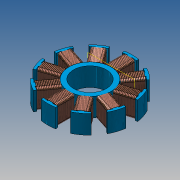
# Autodesk Inventor part: Coil
Saved by Autodesk Inventor 2015 (Build 190159000, 159)
## iProperties
Created: 2016-12-08
Part Number: Coil
Material: Allgemein
Document SubType Name: Modeling
Designer: NS
Density: 1 g/cm^3
Appearance: Default
RuleStatus: InUse
BeforeDocSave0: file://C:\_Vault_ausgecheckt\ilogic\ipt
Author: NS
Autodesk Inventor part; units mm, degrees
ref_plane "YZ Plane" through (0, 0, 0) normal (1, 0, 0) x (0, 1, 0)
ref_plane "XY Plane" through (0, 0, 0) normal (0, 0, 1) x (1, 0, 0)
sketch "Sketch1" plane through (0, 0, 0) normal (0, 0, 1) x (1, 0, 0)
  arc A0 (-1, 8.9443) -> (1, 8.9443) centre (0, 0) ccw
  circle A1 centre (0, 0) radius 7
  line L0 (0, 0) -> (0, 12.6518) construction
  arc A2 (3.1257, 17.7265) -> (0, 18) centre (0, 0) ccw
  arc A3 (0, 18) -> (-3.1257, 17.7265) centre (0, 0) ccw
  arc A4 (-1, 16.9706) -> (-2.952, 16.7417) centre (0, 0) ccw
  arc A5 (2.952, 16.7417) -> (1, 16.9706) centre (0, 0) ccw
  line L1 (-1, 16.9706) -> (-1, 8.9443)
  line L2 (1, 16.9706) -> (1, 8.9443)
  line L3 (-2.952, 16.7417) -> (-3.1257, 17.7265)
  line L4 (2.952, 16.7417) -> (3.1257, 17.7265)
  dimension "d0" = 14
  dimension "d1" = 2
  dimension "d2" = 18
  dimension "d3" = 1
  dimension "d4" = 1
  constraints: 10 end point, 10 point on circle, 6 centre point, 4 symmetric about line, 3 coincident, 2 vertical, 1 point on line, 1 other
  measures "d0" diameter of A1
  measures "d1" radial gap between concentric circles of A0 A1
  measures "d2" radius of A2
  measures "d3" radial gap between concentric circles of A3 A4
  measures "d4" distance between parallel lines of L0 L1
extrude "Extrusion1" add sketch "Sketch1" along normal blind 8
ref_plane "Work Plane1" through (0, 9, 0) normal (0, 1, 0) x (-1, 0, 0)
sketch "Sketch2" plane through (0, 9, 0) normal (0, 1, 0) x (-1, 0, 0)
  line L0 (3.1257, 8) -> (-3.1257, 8) projected
  line L1 (0, 8) -> (0, 0) construction
  line L2 (1.5, 8.225) -> (-1.5, 8.225)
  line L3 (-2.5, 7.225) -> (-2.5, 0.775)
  line L4 (-1.5, -0.225) -> (1.5, -0.225)
  line L5 (2.5, 0.775) -> (2.5, 7.225)
  line L6 (2.5, 8.225) -> (-2.5, -0.225) construction
  line L7 (-2.5, 8.225) -> (2.5, -0.225) construction
  arc A0 (-1.5, 8.225) -> (-2.5, 7.225) centre (-1.5, 7.225) ccw
  arc A1 (-2.5, 0.775) -> (-1.5, -0.225) centre (-1.5, 0.775) ccw
  arc A2 (1.5, -0.225) -> (2.5, 0.775) centre (1.5, 0.775) ccw
  arc A3 (2.5, 7.225) -> (1.5, 8.225) centre (1.5, 7.225) ccw
  point P0 (0, 4)
  dimension "d10" = 5
  dimension "d11" = 8.45
  dimension "d12" = 1
  constraints: 14 end point, 8 point on circle, 8 point on line, 8 tangent, 4 centre point, 4 midpoint, 3 equal radius, 2 parallel, 1 horizontal, 1 perpendicular, 1 vertical
  measures "d10" distance of L6.start L7.start
  measures "d11" distance of L7.start L6.end
  measures "d12" radius of A0
sketch "Sketch4" plane through (0, 0, 0) normal (1, 0, 0) x (0, 1, 0)
  circle A0 centre (9.2417, 8) radius 0.25
  line L0 (16.9706, 8) -> (8.9443, 8) projected
  line L1 (16.7417, 0) -> (16.7417, 8) projected
  point P0 (0, 0)
  point P1 (9, 8.225)
  point P2 (9, 8.225)
  point P3 (9, 8.225)
  dimension "d15" = 0
  dimension "d18" = 0.5
  dimension "d19" = 7.5
  constraints: 1 centre point
  measures "d15" distance from line of L0 A0.centre
  measures "d18" diameter of A0
  measures "d19" distance from line of L1 A0.centre
sweep "Sweep1" add profiles "Sketch4" path "Sketch2" path curves L2 A0 L3 A1 L4 A2 L5 A3
pattern_linear "Rectangular Pattern1" count 15 spacing 0.51 along (0, 1, 0) of "Sweep1"
pattern_circular "Circular Pattern1" count 10 over 360 about axis through (0, 0, 0) along (0, 0, 1) of "Extrusion1", "Sweep1", "Rectangular Pattern1"
body "Solid1"
